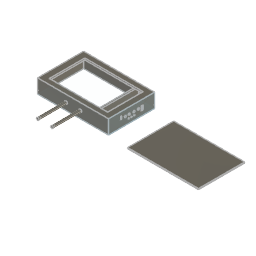
FPV_GROUND_STATION_CAD_CASE (Autodesk Fusion 360 design; units mm, degrees)
part number: 2026-05-24-15-09-10-077
Autodesk Fusion 360 part; units mm, degrees
sketch "Sketch1" plane through (0, 0, 0) normal (0, 0, 1) x (1, 0, 0)
  line L0 (99.4684, -52.4738) -> (-100.5316, -52.4738)
  line L1 (-100.5316, -52.4738) -> (-100.5316, 77.5262)
  line L2 (-100.5316, 77.5262) -> (99.4684, 77.5262)
  line L3 (99.4684, 77.5262) -> (99.4684, -52.4738)
  dimension "d1" = 200
  dimension "d2" = 130
  constraint horizontal L0
  constraint vertical L1
  constraint horizontal L2
  constraint vertical L3
  measures "d1" distance of L0.start L0.end
  measures "d2" distance of L0.start L2.end
extrude "Extrude1" add sketch "Sketch1" along normal blind 40 makes body 1
sketch "Sketch2" plane through (0, 0, 40) normal (0, 0, 1) x (-1, 0, 0)
  line L0 (-99.4684, -77.5262) -> (100.5316, -77.5262)
  line L1 (100.5316, -77.5262) -> (100.5316, 52.4738)
  line L2 (100.5316, 52.4738) -> (-99.4684, 52.4738)
  line L3 (-99.4684, 52.4738) -> (-99.4684, -77.5262)
  line L4 (82, -62.5) -> (-82, -62.5)
  line L5 (-82, -62.5) -> (-82, 37.5)
  line L6 (-82, 37.5) -> (82, 37.5)
  line L7 (82, 37.5) -> (82, -62.5)
  line L8 (82, -62.5) -> (-82, 37.5) construction
  line L9 (-82, -62.5) -> (82, 37.5) construction
  point P0 (0, -12.5)
  dimension "d5" = 164
  dimension "d6" = 100
  constraint horizontal L4
  constraint perpendicular L4 L5
  constraint parallel L4 L6
  constraint parallel L5 L7
  constraint coincident L8 P0
  constraint coincident L9 P0
  measures "d5" distance of L5.end L6.end
  measures "d6" distance of L4.end L5.end
extrude "Extrude2" cut sketch "Sketch2" along normal blind 0 and the other way blind 5 contours L4 L5 L6 L7 bodies 1
sketch "Sketch3" plane through (0, 0, 0) normal (0, 0, -1) x (1, 0, 0)
  line L0 (-100.5316, -77.5262) -> (99.4684, -77.5262)
  line L1 (99.4684, -77.5262) -> (99.4684, 52.4738)
  line L2 (99.4684, 52.4738) -> (-100.5316, 52.4738)
  line L3 (-100.5316, 52.4738) -> (-100.5316, -77.5262)
sketch "Sketch4" plane through (0, 0, 0) normal (0, 0, -1) x (1, 0, 0)
  line L0 (96.4684, 49.4738) -> (-97.5316, 49.4738)
  line L1 (-97.5316, 49.4738) -> (-97.5316, -74.5262)
  line L2 (-97.5316, -74.5262) -> (96.4684, -74.5262)
  line L3 (96.4684, -74.5262) -> (96.4684, 49.4738)
  line L4 (96.4684, 49.4738) -> (-97.5316, -74.5262) construction
  line L5 (-97.5316, 49.4738) -> (96.4684, -74.5262) construction
  line L6 (99.4684, 52.4738) -> (-100.5316, 52.4738)
  line L7 (-100.5316, 52.4738) -> (-100.5316, -77.5262)
  point P0 (-0.5316, -12.5262)
  dimension "d11" = 194
  dimension "d12" = 124
  dimension "d13" = 3
  dimension "d14" = 3
  constraint horizontal L0
  constraint perpendicular L0 L1
  constraint parallel L0 L2
  constraint parallel L1 L3
  constraint coincident L4 P0
  constraint coincident L5 P0
  measures "d11" distance of L1.end L2.end
  measures "d12" distance of L0.end L1.end
  measures "d13" distance of L0 L6
  measures "d14" distance of L1 L7
extrude "Extrude3" cut sketch "Sketch4" along normal blind 0 and the other way blind 35 bodies 1
sketch "Sketch5" plane through (99.4684, 0, 0) normal (1, 0, 0) x (0, 1, 0)
  line L0 (-52.4738, 0) -> (77.5262, 0)
  line L1 (77.5262, 0) -> (77.5262, 40)
  line L2 (77.5262, 40) -> (-52.4738, 40)
  line L3 (-52.4738, 40) -> (-52.4738, 0)
sketch "Sketch6" plane through (99.4684, 0, 0) normal (1, 0, 0) x (0, 1, 0)
  circle A0 centre (-5, 22) radius 3
  circle A1 centre (6, 22) radius 3
  circle A2 centre (19.493, 21.5017) radius 3
  circle A3 centre (31.5, 22) radius 3
  circle A4 centre (4.7, 12.3) radius 2
  circle A5 centre (12.1, 12.4) radius 2
  circle A6 centre (20.0923, 12.2469) radius 2
  line L0 (-18.0153, 28.5707) -> (-15.3483, 28.5707)
  line L1 (-15.3483, 28.5707) -> (-15.3483, 20.4427)
  line L2 (-15.3483, 20.4427) -> (-18.0153, 20.4427)
  line L3 (-18.0153, 20.4427) -> (-18.0153, 28.5707)
  line L4 (39.4285, 24.5918) -> (39.4285, 25.3538)
  line L5 (39.4285, 25.3538) -> (45.2885, 25.3538)
  line L6 (45.2885, 25.3538) -> (45.2885, 12.7038)
  line L7 (45.2885, 12.7038) -> (39.4285, 12.7038)
  line L8 (39.4285, 12.7038) -> (39.4285, 25.3538)
  dimension "d19" = 6
  dimension "d21" = 6
  dimension "d23" = 6
  dimension "d25" = 6
  dimension "d29" = 4
  dimension "d31" = 4
  dimension "d33" = 4
  dimension "d35" = 2.667
  dimension "d36" = 8.128
  dimension "d39" = 0.762
  dimension "d40" = 5.86
  dimension "d41" = 12.65
  constraint horizontal L0
  constraint vertical L1
  constraint horizontal L2
  constraint vertical L3
  constraint horizontal L5
  constraint vertical L6
  constraint horizontal L7
  constraint vertical L8
  measures "d19" diameter of A0
  measures "d21" diameter of A1
  measures "d23" diameter of A2
  measures "d25" diameter of A3
  measures "d29" diameter of A4
  measures "d31" diameter of A5
  measures "d33" diameter of A6
  measures "d35" distance of L0.start L0.end
  measures "d36" distance of L0.start L2.end
  measures "d39" distance of L4.start L4.end
  measures "d40" distance of L4.end L5.end
  measures "d41" distance of L4.end L7.end
extrude "Extrude4" cut sketch "Sketch6" against normal blind 3 bodies 1
sketch "Sketch7" plane through (0, 0, 0) normal (0, 1, 0) x (1, 0, 0)
sketch "Sketch8" plane through (0, -52.4738, 0) normal (0, -1, 0) x (1, 0, 0)
  line L0 (-100.5316, 0) -> (99.4684, 0)
  line L1 (99.4684, 0) -> (99.4684, 40)
  line L2 (99.4684, 40) -> (-100.5316, 40)
  line L3 (-100.5316, 40) -> (-100.5316, 0)
  circle A0 centre (-20, 20) radius 4
  circle A1 centre (20, 20) radius 4
  dimension "d44" = 8
  dimension "d45" = 8
  measures "d44" diameter of A0
  measures "d45" diameter of A1
extrude "Extrude5" cut sketch "Sketch8" against normal blind 3 contours A0 | A1 bodies 1
sketch "Sketch9" plane through (0, -52.4738, 0) normal (0, -1, 0) x (1, 0, 0)
  circle A0 centre (-20, 20) radius 4
  circle A1 centre (20, 20) radius 4
  line L0 (-100.5316, 0) -> (99.4684, 0)
  line L1 (99.4684, 0) -> (99.4684, 40)
  line L2 (99.4684, 40) -> (-100.5316, 40)
  line L3 (-100.5316, 40) -> (-100.5316, 0)
  circle A2 centre (-20, 20) radius 4
  circle A3 centre (20, 20) radius 4
  constraint concentric A0 A2
  constraint concentric A1 A3
extrude "Extrude6" add sketch "Sketch9" along normal blind 80 separate body contours A0 A2 | A1 A3 makes body 2 at (23.995, -105.8071, 19.8006) makes body 3 at (-16.005, -105.8071, 19.8006)
sketch "Sketch10" plane through (0, -49.4738, 0) normal (0, 1, 0) x (-1, 0, 0)
  circle A0 centre (20, 20) radius 4
  circle A1 centre (-20, 20) radius 4
  line L0 (-96.4684, 0) -> (97.5316, 0)
  line L1 (97.5316, 0) -> (97.5316, 35)
  line L2 (97.5316, 35) -> (-96.4684, 35)
  line L3 (-96.4684, 35) -> (-96.4684, 0)
  circle A2 centre (-20, 20) radius 3
  circle A3 centre (20, 20) radius 3
  dimension "d50" = 6
  dimension "d51" = 6
  constraint concentric A1 A2
  constraint concentric A0 A3
  measures "d50" diameter of A2
  measures "d51" diameter of A3
extrude "Extrude7" cut sketch "Sketch10" against normal blind 78 contours A2 | A3 bodies 2 3
sketch "Sketch11" plane through (0, -52.4738, 0) normal (0, -1, 0) x (1, 0, 0)
  circle A0 centre (-20, 20) radius 4
  circle A1 centre (20, 20) radius 4
  line L0 (-100.5316, 0) -> (99.4684, 0)
  line L1 (99.4684, 0) -> (99.4684, 40)
  line L2 (99.4684, 40) -> (-100.5316, 40)
  line L3 (-100.5316, 40) -> (-100.5316, 0)
  line L4 (52.0412, 12.3894) -> (57.0412, 12.3894)
  line L5 (57.0412, 12.3894) -> (57.0412, 32.3894)
  line L6 (57.0412, 32.3894) -> (52.0412, 32.3894)
  line L7 (52.0412, 32.3894) -> (52.0412, 12.3894)
  dimension "d54" = 5
  dimension "d55" = 20
  constraint horizontal L4
  constraint vertical L5
  constraint horizontal L6
  constraint vertical L7
  measures "d54" distance of L4.start L4.end
  measures "d55" distance of L4.start L6.end
extrude "Extrude8" add sketch "Sketch11" against normal blind 130 contours L4 L5 L6 L7 bodies 1
sketch "Sketch12" plane through (0, 0, 0) normal (0, 0, -1) x (1, 0, 0)
  line L0 (-100.5333, 52.4758) -> (99.4667, 52.4758)
  line L1 (99.4667, 52.4758) -> (99.4667, -77.5242)
  line L2 (99.4667, -77.5242) -> (-100.5333, -77.5242)
  line L3 (-100.5333, -77.5242) -> (-100.5333, 52.4758)
  circle A0 centre (-99, 51) radius 0.5
  circle A1 centre (98, 51) radius 0.5
  circle A2 centre (98, -76) radius 0.5
  circle A3 centre (-99, -75.5) radius 0.5
  dimension "d58" = 200
  dimension "d59" = 130
  dimension "d60" = 1
  dimension "d61" = 1
  dimension "d62" = 1
  dimension "d63" = 1
  constraint horizontal L0
  constraint vertical L1
  constraint horizontal L2
  constraint vertical L3
  measures "d58" distance of L0.start L0.end
  measures "d59" distance of L0.start L2.end
  measures "d60" diameter of A0
  measures "d61" diameter of A1
  measures "d62" diameter of A2
  measures "d63" diameter of A3
extrude "Extrude9" cut sketch "Sketch12" against normal blind 10 contours A0 | A1 | A2 | A3 bodies 1
sketch "Sketch13" plane through (0, 0, 0) normal (0, 0, 1) x (1, 0, 0)
  line L0 (159.2828, -58.8395) -> (359.2828, -58.8395)
  line L1 (359.2828, -58.8395) -> (359.2828, 71.1605)
  line L2 (359.2828, 71.1605) -> (159.2828, 71.1605)
  line L3 (159.2828, 71.1605) -> (159.2828, -58.8395)
  dimension "d66" = 200
  dimension "d67" = 130
  constraint horizontal L0
  constraint vertical L1
  constraint horizontal L2
  constraint vertical L3
  measures "d66" distance of L0.start L0.end
  measures "d67" distance of L0.start L2.end
extrude "Extrude10" add sketch "Sketch13" along normal blind 3 separate body makes body 4
